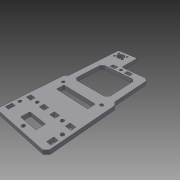
# Autodesk Inventor part: x_carriage_front
Saved by Autodesk Inventor 2014 (Build 180170000, 170)
## iProperties
Created: 2013-11-06
Part Number: x_carriage_front
Material: Generic
Document SubType Name: Modeling
Designer: buben
Density: 1 g/cm^3
Appearance: Anodized - Dark Gray
Author: buben
Subject: Laser Cutted
Autodesk Inventor part; units mm, degrees
ref_plane "YZ Plane" through (0, 0, 0) normal (1, 0, 0) x (0, 1, 0)
ref_plane "XZ Plane" through (0, 0, 0) normal (0, 1, 0) x (-1, 0, 0)
ref_plane "XY Plane" through (0, 0, 0) normal (0, 0, 1) x (1, 0, 0)
sketch "Sketch1" plane through (0, 0, 0) normal (0, 0, 1) x (1, 0, 0)
  line L0 (4, 0) -> (76, 0)
  line L1 (80, 4) -> (80, 87.5)
  line L2 (76, 91.5) -> (4, 91.5)
  line L3 (0, 87.5) -> (0, 4)
  line L4 (0, 4) -> (4, 0)
  line L5 (76, 0) -> (80, 4)
  line L6 (80, 87.5) -> (76, 91.5)
  line L7 (4, 91.5) -> (0, 87.5)
  line L8 (16.5, 75) -> (63.5, 75)
  line L9 (64.5, 74) -> (64.5, 65)
  line L10 (63.5, 64) -> (16.5, 64)
  line L11 (15.5, 65) -> (15.5, 74)
  arc A0 (15.5, 65) -> (16.5, 64) centre (16.5, 65) ccw
  arc A1 (16.5, 75) -> (15.5, 74) centre (16.5, 74) ccw
  arc A2 (64.5, 74) -> (63.5, 75) centre (63.5, 74) ccw
  arc A3 (63.5, 64) -> (64.5, 65) centre (63.5, 65) ccw
  line L12 (28.5, 21) -> (51.5, 21)
  line L13 (52.5, 20) -> (52.5, 11)
  line L14 (51.5, 10) -> (28.5, 10)
  line L15 (27.5, 11) -> (27.5, 20)
  arc A4 (27.5, 11) -> (28.5, 10) centre (28.5, 11) ccw
  arc A5 (28.5, 21) -> (27.5, 20) centre (28.5, 20) ccw
  arc A6 (52.5, 20) -> (51.5, 21) centre (51.5, 20) ccw
  arc A7 (51.5, 10) -> (52.5, 11) centre (51.5, 11) ccw
  line L16 (15.5, 69.5) -> (64.5, 69.5) construction
  line L17 (27.5, 15.5) -> (52.5, 15.5) construction
  circle A8 centre (40, 5) radius 2.25
  circle A9 centre (10, 78.5) radius 2.25
  circle A10 centre (6, 23.25) radius 2.25
  circle A11 centre (74, 23.25) radius 2.25
  circle A12 centre (70, 78.5) radius 2.25
  point P0 (0, 0)
  point P1 (40, 64)
  point P2 (40, 21)
  point P3 (40, 75)
  point P4 (40, 91.5)
  point P5 (0, 45.75)
  point P6 (80, 45.75)
  dimension "d0" = 45
  dimension "d1" = 4
  dimension "d2" = 1
  dimension "d3" = 11
  dimension "d4" = 49
  dimension "d5" = 1
  dimension "d6" = 11
  dimension "d7" = 25
  dimension "d9" = 10
  dimension "d10" = 16.5
  dimension "d11" = 4.5
  dimension "d12" = 4.5
  dimension "d13" = 5
  dimension "d15" = 4.5
  dimension "d16" = 4.5
  dimension "d19" = 54
  dimension "d22" = 80
  dimension "d23" = 6
  dimension "d24" = 6
  dimension "d25" = 23.25
  dimension "d26" = 4.5
  dimension "d27" = 10
  dimension "d28" = 10
  dimension "d54" = 3.5
  constraints: 36 end point, 16 point on circle, 16 tangent, 13 centre point, 10 midpoint, 10 vertical alignment, 8 horizontal alignment, 8 parallel, 4 perpendicular, 3 horizontal
  measures "d0" angle of L0 L4
  measures "d1" horizontal distance of L0.start L3.end
  measures "d2" radius of A1
  measures "d3" distance of L10.start L8.end
  measures "d4" distance of L11.end L9.start
  measures "d5" radius of A5
  measures "d6" distance of L14.start L12.end
  measures "d7" distance of L15.end L13.start
  measures "d9" distance from line of L0 L14.end
  measures "d10" distance from line of L2 L8.start
  measures "d11" diameter of A8
  measures "d12" diameter of A9
  measures "d13" distance from line of L0 A8.centre
  measures "d15" diameter of A10
  measures "d16" diameter of A11
  measures "d19" distance between parallel lines of L17 L16
  measures "d22" distance between parallel lines of L3 L1
  measures "d23" distance from line of L3 A10.centre
  measures "d24" distance from line of L1 A11.centre
  measures "d25" distance from line of L0 A10.centre
  measures "d26" diameter of A12
  measures "d27" distance from line of L3 A9.centre
  measures "d28" distance from line of L1 A12.centre
  measures "d54" distance from line of L8 A9.centre
extrude "Extrusion2" add sketch "Sketch1" along normal blind 6
sketch "Sketch2" plane through (0, 0, 6) normal (0, 0, 1) x (1, 0, 0)
  line L0 (4, 0) -> (76, 0) projected
  circle A0 centre (20, 35) radius 2.25
  circle A1 centre (60, 35) radius 2.25
  line L1 (20, 35) -> (60, 35) construction
  point P0 (0, 0)
  point P1 (40, 35)
  point P2 (40, 0)
  dimension "d31" = 4.5
  dimension "d32" = 4.5
  dimension "d33" = 40
  dimension "d34" = 35
  constraints: 2 centre point, 2 end point, 2 midpoint, 1 horizontal alignment, 1 parallel, 1 vertical alignment
  measures "d31" diameter of A1
  measures "d32" diameter of A0
  measures "d33" distance of L1.end L1.start
  measures "d34" distance from line of L0 L1.end
extrude "Extrusion3" cut sketch "Sketch2" against normal through all
sketch "Sketch3" plane through (0, 0, 6) normal (0, 0, 1) x (1, 0, 0)
  circle A0 centre (20, 35) radius 2.25 projected
  circle A1 centre (60, 35) radius 2.25 projected
  line L0 (80, 4) -> (80, 87.5) projected
  line L1 (0, 87.5) -> (0, 4) projected
  line L2 (27.5, 38) -> (35.5, 38)
  line L3 (35.5, 38) -> (35.5, 32)
  line L4 (35.5, 32) -> (27.5, 32)
  line L5 (27.5, 32) -> (27.5, 38)
  line L6 (44.5, 38) -> (52.5, 38)
  line L7 (52.5, 38) -> (52.5, 32)
  line L8 (52.5, 32) -> (44.5, 32)
  line L9 (44.5, 32) -> (44.5, 38)
  line L10 (67.5, 38) -> (75.5, 38)
  line L11 (75.5, 38) -> (75.5, 32)
  line L12 (75.5, 32) -> (67.5, 32)
  line L13 (67.5, 32) -> (67.5, 38)
  line L14 (4.5, 38) -> (12.5, 38)
  line L15 (12.5, 38) -> (12.5, 32)
  line L16 (12.5, 32) -> (4.5, 32)
  line L17 (4.5, 32) -> (4.5, 38)
  line L18 (3, 16) -> (9, 16)
  line L19 (9, 16) -> (9, 8)
  line L20 (9, 8) -> (3, 8)
  line L21 (3, 8) -> (3, 16)
  line L22 (71, 16) -> (77, 16)
  line L23 (77, 16) -> (77, 8)
  line L24 (77, 8) -> (71, 8)
  line L25 (71, 8) -> (71, 16)
  point P0 (0, 0)
  point P1 (12.5, 35)
  dimension "d37" = 6
  dimension "d38" = 8
  dimension "d39" = 8
  dimension "d40" = 8
  dimension "d41" = 8
  dimension "d42" = 6
  dimension "d43" = 8
  dimension "d44" = 6
  dimension "d45" = 3
  dimension "d46" = 3
  dimension "d47" = 4
  dimension "d48" = 15
  dimension "d49" = 15
  dimension "d50" = 7.5
  dimension "d51" = 7.5
  constraints: 48 end point, 12 parallel, 8 collinear, 6 horizontal, 6 perpendicular, 1 horizontal alignment, 1 midpoint
  measures "d37" distance of L16.end L14.start
  measures "d38" distance of L14.start L14.end
  measures "d39" distance of L2.start L2.end
  measures "d40" distance of L6.start L6.end
  measures "d41" distance of L10.start L10.end
  measures "d42" distance of L18.start L18.end
  measures "d43" distance of L20.end L18.start
  measures "d44" distance of L22.start L22.end
  measures "d45" distance between parallel lines of L1 L21
  measures "d46" distance between parallel lines of L0 L23
  measures "d47" distance from line of L1.end L20
  measures "d48" distance of L2.start L14.end
  measures "d49" distance between parallel lines of L13 L7
  measures "d50" distance from line of A0.centre L15
  measures "d51" distance from line of A1.centre L7
extrude "Extrusion4" cut sketch "Sketch3" against normal through all contours L2 L3 L4 L5 | L6 L7 L8 L9 | L10 L11 L12 L13 | L14 L15 L16 L17 | L18 L19 L20 L21 | L22 L23 L24 L25
sketch "Sketch4" plane through (0, 0, 6) normal (0, 0, 1) x (1, 0, 0)
  line L0 (4, 91.5) -> (76, 91.5)
  line L1 (76, 91.5) -> (76, 151.5)
  line L2 (36, 183.5) -> (4, 183.5)
  line L3 (4, 183.5) -> (4, 91.5)
  line L4 (36, 183.5) -> (36, 151.5)
  line L5 (36, 151.5) -> (76, 151.5)
  point P0 (0, 0)
  dimension "d55" = 92
  dimension "d57" = 32
  dimension "d58" = 32
  constraints: 12 end point, 3 parallel, 2 perpendicular, 1 horizontal
  measures "d55" distance of L2.end L0.start
  measures "d57" distance between parallel lines of L3 L4
  measures "d58" distance of L2.start L4.end
extrude "Extrusion5" add sketch "Sketch4" against normal blind 6
chamfer "Chamfer1" distance 4 angle 45 1 edges at (76, 151.5, 3)
chamfer "Chamfer2" distance 2 angle 45 3 edges at (36, 151.5, 3) (36, 183.5, 3) (4, 183.5, 3)
sketch "Sketch5" plane through (0, 0, 6) normal (0, 0, 1) x (1, 0, 0)
  line L0 (4, 181.5) -> (4, 91.5) projected
  line L1 (34, 183.5) -> (6, 183.5) projected
  line L2 (10, 177.5) -> (24, 177.5) construction
  line L3 (24, 177.5) -> (24, 167.5) construction
  line L4 (24, 167.5) -> (10, 167.5) construction
  line L5 (10, 167.5) -> (10, 177.5) construction
  line L6 (15, 178.5) -> (19, 178.5)
  line L7 (23, 174.5) -> (23, 170.5)
  line L8 (19, 166.5) -> (15, 166.5)
  line L9 (11, 170.5) -> (11, 174.5)
  line L10 (11, 170.5) -> (15, 166.5)
  line L11 (19, 166.5) -> (23, 170.5)
  line L12 (23, 174.5) -> (19, 178.5)
  line L13 (15, 178.5) -> (11, 174.5)
  circle A0 centre (10, 177.5) radius 1.6
  circle A1 centre (10, 167.5) radius 1.6
  circle A2 centre (24, 167.5) radius 1.6
  circle A3 centre (24, 177.5) radius 1.6
  point P0 (0, 0)
  point P1 (23, 172.5)
  point P2 (24, 172.5)
  dimension "d67" = 45
  dimension "d68" = 4
  dimension "d69" = 3.2
  dimension "d70" = 14
  dimension "d71" = 10
  dimension "d72" = 1
  dimension "d73" = 1
  dimension "d74" = 6
  dimension "d75" = 6
  constraints: 24 end point, 9 perpendicular, 4 centre point, 4 coincident, 4 parallel, 3 equal radius, 2 horizontal, 2 midpoint, 1 horizontal alignment
  measures "d67" angle of L10 L8
  measures "d68" distance of L8.start L8.end
  measures "d69" diameter of A1
  measures "d70" distance of L3.end L4.end
  measures "d71" distance of L4.end L2.start
  measures "d72" distance between parallel lines of L5 L9
  measures "d73" distance between parallel lines of L3 L7
  measures "d74" distance between parallel lines of L0 L5
  measures "d75" distance between parallel lines of L1 L2
extrude "Extrusion6" cut sketch "Sketch5" against normal through all
sketch "Sketch6" plane through (0, 0, 6) normal (0, 0, 1) x (1, 0, 0)
  line L0 (72, 151.5) -> (38, 151.5) projected
  line L1 (16.5, 75) -> (63.5, 75) projected
  line L2 (24.5, 148.5) -> (32.5, 148.5)
  line L3 (32.5, 148.5) -> (32.5, 142.5)
  line L4 (32.5, 142.5) -> (24.5, 142.5)
  line L5 (24.5, 142.5) -> (24.5, 148.5)
  line L6 (47.5, 148.5) -> (55.5, 148.5)
  line L7 (55.5, 148.5) -> (55.5, 142.5)
  line L8 (55.5, 142.5) -> (47.5, 142.5)
  line L9 (47.5, 142.5) -> (47.5, 148.5)
  line L10 (32.5, 148.5) -> (47.5, 142.5) construction
  line L11 (47.5, 148.5) -> (32.5, 142.5) construction
  circle A0 centre (40, 145.5) radius 2.25
  point P0 (0, 0)
  point P1 (40, 75)
  dimension "d78" = 6
  dimension "d79" = 8
  dimension "d80" = 8
  dimension "d81" = 15
  dimension "d82" = 4.5
  dimension "d83" = 3
  constraints: 20 end point, 4 parallel, 2 collinear, 2 horizontal, 2 midpoint, 2 perpendicular, 1 centre point, 1 vertical alignment
  measures "d78" distance of L4.end L2.start
  measures "d79" distance of L2.start L2.end
  measures "d80" distance of L6.start L6.end
  measures "d81" distance between parallel lines of L3 L9
  measures "d82" diameter of A0
  measures "d83" distance between parallel lines of L0 L6
extrude "Extrusion7" cut sketch "Sketch6" against normal through all
sketch "Sketch7" plane through (0, 0, 6) normal (0, 0, 1) x (1, 0, 0)
  line L0 (32.5, 142.5) -> (24.5, 142.5) projected
  line L1 (4, 181.5) -> (4, 91.5) projected
  line L2 (76, 91.5) -> (76, 147.5) projected
  line L3 (18, 139.5) -> (62, 139.5)
  line L4 (66, 135.5) -> (66, 95.5)
  line L5 (62, 91.5) -> (18, 91.5)
  line L6 (14, 95.5) -> (14, 135.5)
  line L7 (14, 135.5) -> (18, 139.5)
  line L8 (14, 95.5) -> (18, 91.5)
  line L9 (62, 91.5) -> (66, 95.5)
  line L10 (66, 135.5) -> (62, 139.5)
  point P0 (0, 0)
  point P1 (14, 139.5)
  point P2 (66, 91.5)
  point P3 (66, 139.5)
  point P4 (14, 91.5)
  dimension "d86" = 4
  dimension "d87" = 4
  dimension "d88" = 4
  dimension "d89" = 4
  dimension "d90" = 4
  dimension "d91" = 4
  dimension "d92" = 4
  dimension "d93" = 4
  dimension "d94" = 10
  dimension "d95" = 10
  dimension "d96" = 3
  constraints: 16 end point, 8 point on line, 2 parallel, 1 horizontal, 1 horizontal alignment, 1 perpendicular
  measures "d86" distance of L6.end point (14, 139.5)
  measures "d87" distance of L3.start point (14, 139.5)
  measures "d88" distance of L6.start point (14, 91.5)
  measures "d89" distance of L5.end point (14, 91.5)
  measures "d90" distance of L5.start point (66, 91.5)
  measures "d91" distance of L4.end point (66, 91.5)
  measures "d92" distance of L4.start point (66, 139.5)
  measures "d93" distance of L3.end point (66, 139.5)
  measures "d94" distance between parallel lines of L1 L6
  measures "d95" distance between parallel lines of L2 L4
  measures "d96" distance between parallel lines of L3 L0
extrude "Extrusion8" cut sketch "Sketch7" against normal through all
equation "\"d87\" = d86"
equation "\"d88\" = d86"
equation "\"d89\" = d88"
equation "\"d90\" = d86"
equation "\"d91\" = d90"
equation "\"d92\" = d86"
equation "\"d93\" = d92"
equation "\"d95\" = d94"
body "Solid2"
